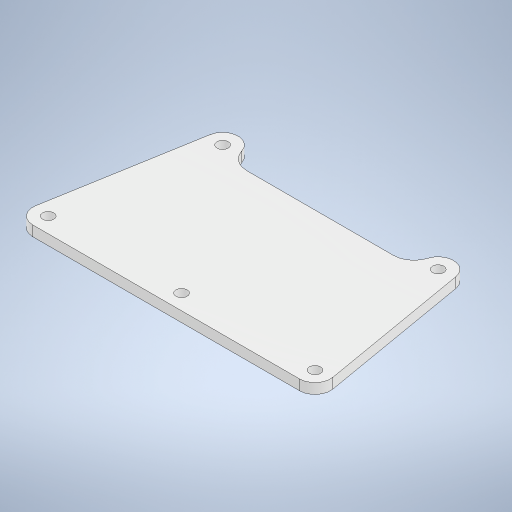
# Autodesk Inventor part: Pod
Saved by Autodesk Inventor 2023.2 (Build 272271000, 271)
## iProperties
Created: 2023-06-26
Part Number: Pod
Material: UHMW, White
Document SubType Name: Modeling
Designer: Nathan Cai
Density: 0.94 g/cm^3
Appearance: Smooth - White
Mass: 19 g
Surface Area: 229.905 cm^2
Volume: 60.4978 cm^3
Author: Nathan Cai
Autodesk Inventor part; units mm, degrees
ref_plane "YZ Plane" through (0, 0, 0) normal (1, 0, 0) x (0, 1, 0)
ref_plane "XZ Plane" through (0, 0, 0) normal (0, 1, 0) x (-1, 0, 0)
ref_plane "XY Plane" through (0, 0, 0) normal (0, 0, 1) x (1, 0, 0)
sketch "Sketch22" plane through (0, 0, 0) normal (0, 1, 0) x (-1, 0, 0)
  circle A0 centre (0, 0) radius 1.7526
  line L0 (0, 0) -> (-41.275, 0) construction
  circle A1 centre (-41.275, 0) radius 1.7526
  circle A2 centre (-82.55, -15.875) radius 1.7526
  circle A3 centre (-33.3375, -46.0375) radius 1.7526
  circle A4 centre (-34.925, -69.85) radius 1.7526
  circle A5 centre (-76.2, -55.5625) radius 1.7526
  circle A6 centre (-38.1, -87.3125) radius 3.302 construction
  circle A7 centre (-52.7601, -77.7875) radius 3.175 construction
  circle A8 centre (-76.2, -55.5625) radius 6.35 construction
  circle A9 centre (-38.1, -87.3125) radius 9.525 construction
  line L1 (-44.6537, -94.2244) -> (-85.429, -55.5625)
  line L2 (-46.8012, -83.4376) -> (-71.592, -59.9316) construction
  line L3 (-71.4375, -49.2125) -> (-88.9, -49.2125)
  line L4 (-88.9, -49.2125) -> (-88.9, -20.6375) construction
  line L5 (-88.9, -20.6375) -> (-71.4375, -20.6375)
  line L6 (-71.4375, -20.6375) -> (-71.4375, -49.2125)
  line L7 (-88.9, -49.2125) -> (-82.55, -49.2125)
  line L8 (-82.55, -49.2125) -> (-82.55, -55.5625) construction
  line L9 (-82.55, -55.5625) -> (-88.9, -55.5625)
  line L10 (-88.9, -55.5625) -> (-88.9, -49.2125)
  line L11 (-28.575, -87.3125) -> (-28.575, -42.8625)
  line L12 (-35.0901, -42.8625) -> (0, -42.8625)
  line L13 (0, -42.8625) -> (0, -38.1) construction
  line L14 (0, -38.1) -> (-35.0901, -38.1)
  line L15 (-35.0901, -38.1) -> (-35.0901, -42.8625) construction
  line L16 (-73.025, 4.7625) -> (0, 4.7625)
  line L17 (0, 4.7625) -> (0, -4.7625) construction
  line L18 (0, -4.7625) -> (-73.025, -4.7625)
  line L19 (-73.025, -4.7625) -> (-73.025, 4.7625)
  line L20 (-73.025, 4.7625) -> (0, -4.7625) construction
  line L21 (0, 4.7625) -> (-73.025, -4.7625) construction
  line L22 (-88.9, -20.6375) -> (-73.025, -20.6375)
  line L23 (-73.025, -20.6375) -> (-73.025, 0) construction
  line L24 (-73.025, 0) -> (-88.9, 0)
  line L25 (-88.9, 0) -> (-88.9, -20.6375)
  circle A10 centre (-52.7601, -77.7875) radius 6.35 construction
  circle A11 centre (-34.925, -69.85) radius 6.35 construction
  line L26 (-28.575, -74.7551) -> (-57.283, -82.2497)
  circle A12 centre (-33.3375, -46.0375) radius 4.7625
  arc A13 (-40.4658, -4.6933) -> (-45.9683, -0.8092) centre (-41.275, 0) ccw
  line L27 (-33.3375, -46.0375) -> (-41.275, 0) construction
  circle A14 centre (-82.55, -15.875) radius 4.7625
  line L28 (-42.9846, 4.4451) -> (-84.2596, -11.4299)
  line L29 (-87.3125, -15.875) -> (-87.3125, -20.6375)
  circle A15 centre (0, 0) radius 1.7526
  line L30 (0, 0) -> (41.275, 0) construction
  circle A16 centre (41.275, 0) radius 1.7526
  circle A17 centre (82.55, -15.875) radius 1.7526
  circle A18 centre (33.3375, -46.0375) radius 1.7526
  circle A19 centre (34.925, -69.85) radius 1.7526
  circle A20 centre (76.2, -55.5625) radius 1.7526
  circle A21 centre (38.1, -87.3125) radius 3.302 construction
  circle A22 centre (52.7601, -77.7875) radius 3.175 construction
  circle A23 centre (76.2, -55.5625) radius 6.35 construction
  circle A24 centre (38.1, -87.3125) radius 9.525 construction
  line L31 (44.6537, -94.2244) -> (85.429, -55.5625)
  line L32 (46.8012, -83.4376) -> (71.592, -59.9316) construction
  line L33 (71.4375, -49.2125) -> (88.9, -49.2125)
  line L34 (88.9, -49.2125) -> (88.9, -20.6375) construction
  line L35 (88.9, -20.6375) -> (71.4375, -20.6375)
  line L36 (71.4375, -20.6375) -> (71.4375, -49.2125)
  line L37 (88.9, -49.2125) -> (82.55, -49.2125)
  line L38 (82.55, -49.2125) -> (82.55, -55.5625) construction
  line L39 (82.55, -55.5625) -> (88.9, -55.5625)
  line L40 (88.9, -55.5625) -> (88.9, -49.2125)
  line L41 (28.575, -87.3125) -> (28.575, -42.8625)
  line L42 (35.0901, -42.8625) -> (0, -42.8625)
  line L43 (0, -38.1) -> (35.0901, -38.1)
  line L44 (35.0901, -38.1) -> (35.0901, -42.8625) construction
  line L45 (73.025, 4.7625) -> (0, 4.7625)
  line L46 (0, -4.7625) -> (73.025, -4.7625)
  line L47 (73.025, -4.7625) -> (73.025, 4.7625)
  line L48 (73.025, 4.7625) -> (0, -4.7625) construction
  line L49 (0, 4.7625) -> (73.025, -4.7625) construction
  line L50 (88.9, -20.6375) -> (73.025, -20.6375)
  line L51 (73.025, -20.6375) -> (73.025, 0) construction
  line L52 (73.025, 0) -> (88.9, 0)
  line L53 (88.9, 0) -> (88.9, -20.6375)
  circle A25 centre (52.7601, -77.7875) radius 6.35 construction
  circle A26 centre (34.925, -69.85) radius 6.35 construction
  line L54 (28.575, -74.7551) -> (57.283, -82.2497)
  circle A27 centre (33.3375, -46.0375) radius 4.7625
  arc A28 (45.9683, -0.8092) -> (40.4658, -4.6933) centre (41.275, 0) ccw
  line L55 (33.3375, -46.0375) -> (41.275, 0) construction
  circle A29 centre (82.55, -15.875) radius 4.7625
  line L56 (42.9846, 4.4451) -> (84.2596, -11.4299)
  line L57 (87.3125, -15.875) -> (87.3125, -20.6375)
  circle A30 centre (-52.7601, -77.7875) radius 1.7526
  circle A31 centre (52.7601, -77.7875) radius 1.7526
  circle A32 centre (-33.3375, -46.0375) radius 3.175 construction
  line L58 (38.0308, -46.8467) -> (45.9683, -0.8092)
  line L59 (-38.0308, -46.8467) -> (-45.9683, -0.8092)
  point P0 (-36.5125, 0)
  point P1 (-57.2791, -82.2486)
  point P2 (36.5125, 0)
  point P3 (57.2791, -82.2486)
  point P4 (-41.275, 4.7625)
  point P5 (41.275, 4.7625)
  point P6 (-33.8849, -42.8625)
  point P7 (-33.3375, -44.2849)
  point P8 (-33.6353, -44.3104)
  point P9 (33.3375, -44.2849)
  point P10 (33.8849, -42.8625)
  point P11 (33.6353, -44.3104)
  point P12 (40.4539, -4.7625)
  point P13 (34.706, -38.1)
  point P14 (-34.706, -38.1)
  point P15 (-40.4539, -4.7625)
  point P16 (-28.575, -46.0375)
  point P17 (28.575, -46.0375)
  dimension "d151" = 3.5052
  dimension "d152" = 41.275
  dimension "d153" = 3.5052
  dimension "d154" = 3.5052
  dimension "d155" = 15.875
  dimension "d156" = 41.275
  dimension "d157" = 3.5052
  dimension "d158" = 7.9375
  dimension "d159" = 46.0375
  dimension "d160" = 3.5052
  dimension "d161" = 6.35
  dimension "d162" = 69.85
  dimension "d163" = 3.5052
  dimension "d164" = 34.925
  dimension "d165" = 55.5625
  dimension "d166" = 6.604
  dimension "d167" = 87.3125
  dimension "d168" = 38.1
  dimension "d169" = 6.35
  dimension "d170" = 12.7
  dimension "d171" = 19.05
  dimension "d172" = 6.35
  dimension "d173" = 9.525
  dimension "d174" = 49.2125
  dimension "d175" = 28.575
  dimension "d176" = 4.7625
  dimension "d177" = 88.9
  dimension "d178" = 6.35
  dimension "d179" = 4.7625
  dimension "d180" = 9.525
  dimension "d181" = 73.025
  dimension "d182" = 3.5052
  dimension "d183" = 3.5052
  dimension "d187" = 6.35
  constraints: 120 end point, 44 symmetric about line, 30 centre point, 20 coincident, 20 point on circle, 19 point on line, 15 tangent, 11 parallel, 7 perpendicular, 6 horizontal, 4 midpoint, 2 vertical, 25 other
  measures "d151" diameter of A0
  measures "d152" distance of L0.start L0.end
  measures "d153" diameter of A1
  measures "d154" diameter of A2
  measures "d155" vertical distance of A1.centre A2.centre
  measures "d156" horizontal distance of A1.centre A2.centre
  measures "d157" diameter of A3
  measures "d158" horizontal distance of A1.centre A3.centre
  measures "d159" vertical distance of A1.centre A3.centre
  measures "d160" diameter of A4
  measures "d161" horizontal distance of A1.centre A4.centre
  measures "d162" vertical distance of A1.centre A4.centre
  measures "d163" diameter of A5
  measures "d164" horizontal distance of A1.centre A5.centre
  measures "d165" vertical distance of A1.centre A5.centre
  measures "d166" diameter of A6
  measures "d167" vertical distance of L0.start A6.centre
  measures "d168" horizontal distance of L0.start A6.centre
  measures "d169" diameter of A7
  measures "d170" diameter of A8
  measures "d171" diameter of A9
  measures "d172" distance between parallel lines of L1 L2
  measures "d173" vertical distance of A7.centre A6.centre
  measures "d174" distance from line of L0.start L3
  measures "d175" distance between parallel lines of L5 L3
  measures "d176" distance from line of A5.centre L6
  measures "d177" distance from line of L0.start L4
  measures "d178" distance between parallel lines of L3 L9
  measures "d179" distance of L13.end L12.end
  measures "d180" distance between parallel lines of L16 L18
  measures "d181" distance between parallel lines of L17 L19
  measures "d182" diameter of A30
  measures "d183" diameter of A31
  measures "d187" diameter of A32
extrude "Extrusion20" add sketch "Sketch22" along normal blind 3.175 contours A12 L12 L11 | A12 | L12 A12 L59 L18 L46 L58 A27 L42 | L59 A13 L16 L45 A28 L58 L46 L18 | L42 A27 L41 | A27
fillet "Fillet13" radius 6.35 2 edges at (28.575, 1.5875, -42.8625) (-28.575, 1.5875, -42.8625)
body "Solid2"
